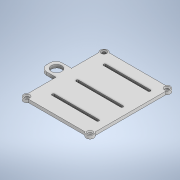
# Autodesk Inventor part: Part2
Saved by Autodesk Inventor 2021 (Build 250183000, 183)
## iProperties
Created: 2021-09-30
Part Number: Part2
Material: Generic
Document SubType Name: Modeling
Designer: david
Density: 1 g/cm^3
Appearance: Default
Author: david
## iProperties of the stored document _3DPrint.ipt
Created: 2021-09-30
Part Number: _3DPrint
Material: Generic
Document SubType Name: Modeling
Designer: david
Density: 1 g/cm^3
Appearance: Default
Author: david
Autodesk Inventor part; units mm, degrees
ref_plane "YZ Plane" through (0, 0, 0) normal (1, 0, 0) x (0, 1, 0)
ref_plane "XZ Plane" through (0, 0, 0) normal (0, 1, 0) x (-1, 0, 0)
ref_plane "XY Plane" through (0, 0, 0) normal (0, 0, 1) x (1, 0, 0)
sketch "Sketch1" plane through (0, 0, 0) normal (0, 1, 0) x (-1, 0, 0)
  line L0 (-32.25, -38.75) -> (32.25, -38.75)
  line L1 (32.25, -38.75) -> (32.25, 38.75)
  line L2 (32.25, 38.75) -> (-32.25, 38.75)
  line L3 (-32.25, 38.75) -> (-32.25, -38.75)
  line L4 (-32.25, -38.75) -> (32.25, 38.75) construction
  line L5 (32.25, -38.75) -> (-32.25, 38.75) construction
  point P0 (0, 0)
  dimension "d0" = 64.5
  dimension "d1" = 77.5
  constraints: 12 end point, 2 midpoint, 2 parallel, 1 horizontal, 1 perpendicular
  measures "d0" distance of L2.end L1.end
  measures "d1" distance of L1.end L0.end
extrude "Extrusion1" add sketch "Sketch1" along normal blind 3
sketch "Sketch4" plane through (-32.25, 0, -38.75) normal (-1, 0, 0) x (0, 0, 1)
  line L0 (0, 3) -> (77.5, 3) projected
  line L1 (0, 0) -> (77.5, 0) projected
  line L2 (31, 3) -> (46, 3)
  line L3 (46, 3) -> (46, 0)
  line L4 (46, 0) -> (31, 0)
  line L5 (31, 0) -> (31, 3)
  line L6 (0, 0) -> (0, 3) projected
  line L7 (77.5, 0) -> (77.5, 3) projected
  point P0 (38.75, 0)
  dimension "d17" = 15
  dimension "d18" = 31
  dimension "d19" = 31.5
  constraints: 8 end point, 2 parallel, 2 point on line, 1 horizontal, 1 perpendicular
  measures "d17" distance of L3.end L4.end
  measures "d18" distance between parallel lines of L6 L5
  measures "d19" distance between parallel lines of L7 L3
extrude "Extrusion3" add sketch "Sketch4" along normal blind 15 contours L0 L3 L1 L5
sketch "Sketch5" plane through (0, 3, 0) normal (0, 1, 0) x (1, 0, 0)
  circle A0 centre (-39.25, 0.25) radius 5
  line L0 (-32.25, -7.25) -> (-47.25, -7.25) projected
  line L1 (-32.25, 7.75) -> (-47.25, 7.75) projected
  line L2 (-47.25, -7.25) -> (-47.25, 7.75) projected
  point P0 (0, 0)
  dimension "d22" = 10
  dimension "d34" = 7.5
  dimension "d35" = 7.5
  dimension "d36" = 8
  constraints: 1 centre point
  measures "d22" diameter of A0
  measures "d34" distance from line of L0 A0.centre
  measures "d35" distance from line of L1 A0.centre
  measures "d36" distance from line of L2 A0.centre
extrude "Extrusion4" cut sketch "Sketch5" against normal up to surface (3 mm away)
fillet "Fillet1" radius 6 2 edges at (-47.25, 1.5, 7.25) (-47.25, 1.5, -7.75)
sketch "Sketch6" plane through (0, 0, 0) normal (0, -1, 0) x (1, 0, 0)
  line L0 (-19.1342, -27.716) -> (23.9028, -27.716)
  line L1 (24.9028, -26.716) -> (24.9028, -26.3695)
  line L2 (23.9028, -25.3695) -> (-19.1342, -25.3695)
  line L3 (-20.1342, -26.3695) -> (-20.1342, -26.716)
  arc A0 (-20.1342, -26.716) -> (-19.1342, -27.716) centre (-19.1342, -26.716) ccw
  arc A1 (-19.1342, -25.3695) -> (-20.1342, -26.3695) centre (-19.1342, -26.3695) ccw
  arc A2 (23.9028, -27.716) -> (24.9028, -26.716) centre (23.9028, -26.716) ccw
  arc A3 (24.9028, -26.3695) -> (23.9028, -25.3695) centre (23.9028, -26.3695) ccw
  line L4 (-19.1342, -1.2568) -> (23.9028, -1.2568)
  line L5 (24.9028, -0.2568) -> (24.9028, 0.0896)
  line L6 (23.9028, 1.0896) -> (-19.1342, 1.0896)
  line L7 (-20.1342, 0.0896) -> (-20.1342, -0.2568)
  arc A4 (-20.1342, -0.2568) -> (-19.1342, -1.2568) centre (-19.1342, -0.2568) ccw
  arc A5 (-19.1342, 1.0896) -> (-20.1342, 0.0896) centre (-19.1342, 0.0896) ccw
  arc A6 (23.9028, -1.2568) -> (24.9028, -0.2568) centre (23.9028, -0.2568) ccw
  arc A7 (24.9028, 0.0896) -> (23.9028, 1.0896) centre (23.9028, 0.0896) ccw
  line L8 (-19.1342, 21.9427) -> (23.9028, 21.9427)
  line L9 (24.9028, 22.9427) -> (24.9028, 23.2892)
  line L10 (23.9028, 24.2892) -> (-19.1342, 24.2892)
  line L11 (-20.1342, 23.2892) -> (-20.1342, 22.9427)
  arc A8 (-20.1342, 22.9427) -> (-19.1342, 21.9427) centre (-19.1342, 22.9427) ccw
  arc A9 (-19.1342, 24.2892) -> (-20.1342, 23.2892) centre (-19.1342, 23.2892) ccw
  arc A10 (23.9028, 21.9427) -> (24.9028, 22.9427) centre (23.9028, 22.9427) ccw
  arc A11 (24.9028, 23.2892) -> (23.9028, 24.2892) centre (23.9028, 23.2892) ccw
  point P0 (0, 0)
  dimension "d27" = 1
  dimension "d28" = 1
  dimension "d29" = 1
  constraints: 24 end point, 24 point on circle, 24 tangent, 12 centre point, 9 equal radius, 6 parallel, 3 horizontal, 3 perpendicular
  measures "d27" radius of A0
  measures "d28" radius of A4
  measures "d29" radius of A8
extrude "Extrusion5" cut sketch "Sketch6" against normal up to surface (3 mm away)
sketch "Sketch7" plane through (0, 3, 0) normal (0, 1, 0) x (1, 0, 0)
  circle A0 centre (-30.232, -37.014) radius 3.5
  line L0 (-32.25, -38.75) -> (32.25, -38.75) projected
  line L1 (-32.25, -7.25) -> (-32.25, -38.75) projected
  circle A1 centre (30.232, -37.014) radius 3.5
  circle A2 centre (-30.232, 37.014) radius 3.5
  circle A3 centre (30.232, 37.014) radius 3.5
  line L2 (32.25, 38.75) -> (-32.25, 38.75) projected
  line L3 (-32.25, 38.75) -> (-32.25, 7.75) projected
  line L4 (32.25, -38.75) -> (32.25, 38.75) projected
  point P0 (0, 0)
  dimension "d37" = 7
  dimension "d38" = 1.736
  dimension "d39" = 2.018
  dimension "d40" = 7
  dimension "d41" = 7
  dimension "d42" = 7
  dimension "d43" = 1.736
  dimension "d44" = 2.018
  dimension "d45" = 1.736
  dimension "d46" = 2.018
  dimension "d47" = 1.736
  dimension "d48" = 2.018
  constraints: 4 centre point
  measures "d37" diameter of A0
  measures "d38" distance from line of L0 A0.centre
  measures "d39" distance from line of L1 A0.centre
  measures "d40" diameter of A1
  measures "d41" diameter of A2
  measures "d42" diameter of A3
  measures "d43" distance from line of L2 A2.centre
  measures "d44" distance from line of L3 A2.centre
  measures "d45" distance from line of L2 A3.centre
  measures "d46" distance from line of L4 A3.centre
  measures "d47" distance from line of L0 A1.centre
  measures "d48" distance from line of L4 A1.centre
extrude "Extrusion6" add sketch "Sketch7" against normal up to surface (3 mm away)
sketch "Sketch8" plane through (0, 3, 0) normal (0, 1, 0) x (1, 0, 0)
  circle A0 centre (30.232, -37.014) radius 1.6
  circle A1 centre (-30.232, -37.014) radius 1.6
  circle A2 centre (-30.232, 37.014) radius 1.6
  circle A3 centre (30.232, 37.014) radius 1.6
  point P0 (0, 0)
  dimension "d51" = 3.2
  dimension "d52" = 3.2
  dimension "d53" = 3.2
  dimension "d54" = 3.2
  constraints: 4 centre point
  measures "d51" diameter of A0
  measures "d52" diameter of A1
  measures "d53" diameter of A2
  measures "d54" diameter of A3
extrude "Extrusion7" cut sketch "Sketch8" against normal up to surface (3 mm away)
chamfer "Chamfer1" distance 1 angle 45 4 edges at (-31.832, 3, 37.014) (28.632, 3, -37.014) (-31.832, 3, -37.014) (28.632, 3, 37.014)
body "Solid1"
